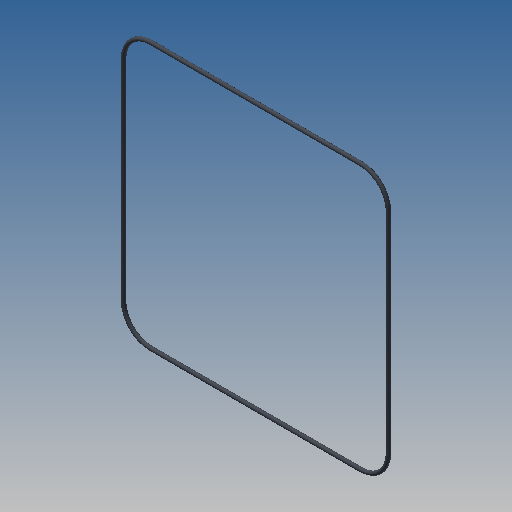
# Autodesk Inventor part: 9452K302
Saved by Autodesk Inventor 2018.2 (Build 222227000, 227)
## iProperties
Created: 2014-04-04
Material: VERO BLACK
Vendor: MCMASTER
Document SubType Name: Modeling
Designer: NEGRASHOVI
Mass: 247.244 g
Surface Area: 1522.49 cm^2
Volume: 211.319 cm^3
Density: 1.17 g/cm^3
Description: O-RING DASH 052
Project: COMMON
Appearance: Black Anodize
Part Number: 9452K302
RuleStatus: InUse
AfterDocSave0: file://Part Number Cleaner
LAB/DEPT: COMMON
REQUESTING SCIENTIST: COMMON
SURFACE ROUGHNESS: N/A
DESIGN DEPARTMENT: HHMI: JRC - ID&F
SPECIAL FINISH: NONE
ALTERED ITEM PART NUMBER: N/A
ALTERED ITEM VENDOR: N/A
ALTERED ITEM DESCRIPTION: N/A
Author: NEGRASHOVI
Revision Number: -
Autodesk Inventor part; units mm, degrees
ref_plane "YZ Plane" through (0, 0, 0) normal (1, 0, 0) x (0, 1, 0)
ref_plane "XZ Plane" through (0, 0, 0) normal (0, 1, 0) x (-1, 0, 0)
ref_plane "XY Plane" through (0, 0, 0) normal (0, 0, 1) x (1, 0, 0)
sketch "Sketch17" plane through (0, 0, 0) normal (0, 0, -1) x (-1, 0, 0)
  line L0 (-47.9679, 60.6679) -> (47.9679, 60.6679)
  line L1 (60.6679, 47.9679) -> (60.6679, -47.9679)
  line L2 (47.9679, -60.6679) -> (-47.9679, -60.6679)
  line L3 (-60.6679, -47.9679) -> (-60.6679, 47.9679)
  arc A0 (-47.9679, 60.6679) -> (-60.6679, 47.9679) centre (-47.9679, 47.9679) ccw
  arc A1 (60.6679, 47.9679) -> (47.9679, 60.6679) centre (47.9679, 47.9679) ccw
  arc A2 (47.9679, -60.6679) -> (60.6679, -47.9679) centre (47.9679, -47.9679) ccw
  arc A3 (-60.6679, -47.9679) -> (-47.9679, -60.6679) centre (-47.9679, -47.9679) ccw
  point P0 (0, 60.6679)
  point P1 (60.6679, 0)
  point P2 (0, 0)
  dimension "d126" = 12.7
  dimension "d127" = 19.9491
  dimension "d128" = 95.9358
  constraints: 8 end point, 8 point on circle, 8 tangent, 4 centre point, 3 equal radius, 2 midpoint, 2 parallel, 2 perpendicular, 1 horizontal, 1 horizontal alignment, 1 vertical alignment
  measures "d126" radius of A0
  measures "d128" distance of L2.start L2.end
sketch "Sketch18" plane through (0, 0, 0) normal (0, 1, 0) x (-1, 0, 0)
  circle A0 centre (-60.6679, 0) radius 0.889
  point P0 (0, 0)
  dimension "d129" = 1.778
  constraints: 1 centre point, 1 coincident
  measures "d129" diameter of A0
sweep "Sweep2" add profiles "Sketch18" path "Sketch17"
body "Solid4"
